FrameCenterServoHolder (Autodesk Fusion 360 design; units mm, degrees)
Autodesk Fusion 360 part; units mm, degrees
sketch "Sketch1" plane through (0, 0, 0) normal (0, 1, 0) x (1, 0, 0)
  line L0 (0, 26) -> (7, 26)
  line L1 (7, 26) -> (7, 6)
  line L2 (7, 6) -> (48, 6)
  line L3 (48, 6) -> (48, 26)
  line L4 (48, 26) -> (55, 26)
  line L5 (55, 26) -> (55, -9.8)
  line L6 (55, -9.8) -> (30.3, -9.8)
  line L7 (30.3, -9.8) -> (20.5, 0)
  line L8 (20.5, 0) -> (0, 0)
  line L9 (0, 26) -> (0, 0)
  line L10 (0, 0) -> (0, 39.3629) construction
  dimension "d1" = 7
  dimension "d2" = 7
  dimension "d3" = 41
  dimension "d4" = 6
  dimension "d5" = 15.8
  dimension "d7" = 135
  dimension "d8" = 20
  dimension "d98" = 20.5
  constraint perpendicular L0 L1
  constraint perpendicular L1 L2
  constraint perpendicular L2 L3
  constraint perpendicular L1 L4
  constraint perpendicular L4 L5
  constraint perpendicular L5 L6
  constraint collinear L0 L4
  constraint coincident L9.end L8
  constraint coincident L8.end L9.end
  constraint perpendicular L8 L9
  constraint vertical L10
  constraint collinear L9 L10
  measures "d1" distance of L0.start L0.end
  measures "d2" distance of L3.end L4.end
  measures "d3" distance of L1 L3
  measures "d4" distance of L2 L8
  measures "d5" distance of L2 L6
  measures "d7" angle of L6 L7
  measures "d8" distance of L2 L4
  measures "d98" distance of L7.end L8.end
extrude "Extrude1" add sketch "Sketch1" along normal blind 16
sketch "Sketch2" plane through (0, 16, 0) normal (0, 1, 0) x (-1, 0, 0)
  line L0 (-7, -26) -> (0, -26)
  line L1 (0, -26) -> (0, 0)
  line L2 (0, 0) -> (-20.5, 0)
  line L3 (-20.5, 0) -> (-30.3, 9.8)
  line L4 (-30.3, 9.8) -> (-55, 9.8)
  line L5 (-55, 9.8) -> (-55, -26)
  line L6 (-55, -26) -> (-48, -26)
  line L7 (-48, -26) -> (-48, -6)
  line L8 (-48, -6) -> (-7, -6)
  line L9 (-7, -6) -> (-7, -26)
  line L10 (-3, -22) -> (-52, -22) construction
  line L11 (-52, -22) -> (-52, -12) construction
  line L12 (-52, -12) -> (-3, -12) construction
  line L13 (-3, -12) -> (-3, -22) construction
  circle A0 centre (-3, -22) radius 1.75
  circle A1 centre (-3, -12) radius 1.75
  circle A2 centre (-52, -22) radius 1.75
  circle A3 centre (-52, -12) radius 1.75
  dimension "d11" = 3.5
  dimension "d12" = 3.5
  dimension "d13" = 3.5
  dimension "d14" = 3.5
  dimension "d15" = 49
  dimension "d16" = 10
  dimension "d17" = 55
  dimension "d18" = 20
  dimension "d19" = 4
  dimension "d20" = 3
  constraint horizontal L10
  constraint vertical L11
  constraint horizontal L12
  constraint vertical L13
  constraint coincident L10.start L13.end
  constraint coincident L12.end L13.start
  constraint coincident L10.end L11.start
  constraint coincident L11.end L12.start
  measures "d11" diameter of A0
  measures "d12" diameter of A1
  measures "d13" diameter of A2
  measures "d14" diameter of A3
  measures "d15" distance of L10.start L10.end
  measures "d16" distance of L10.start L12.end
  measures "d17" distance of L1 L5
  measures "d18" distance of L6.end L7.end
  measures "d19" distance of L6 L10
  measures "d20" distance of L1 L13
extrude "Extrude2" cut sketch "Sketch2" against normal up to surface (16 mm away) contours A0 | A1 | A2 | A3
ref_plane "WorkPlane1" through (27.5, 8, -8.1) normal (0, 1, 0) x (0, 0, 1)
ref_plane "WorkPlane2" through (27.5, 8, -16) normal (0, 0, -1) x (-1, 0, 0)
ref_plane "WorkPlane3" through (27.5, 8, -16) normal (-1, 0, 0) x (0, 0, 1)
ref_plane "WorkPlane4" through (27.5, 8, -8.1) normal (0, 1, 0) x (0, 0, 1)
sketch "Sketch3" plane through (27.5, 8, -7.6) normal (0, 1, 0) x (1, 0, 0)
  circle A0 centre (-24.5, 4.4) radius 1.75
  circle A1 centre (24.5, 14.4) radius 1.75
  circle A2 centre (-24.5, 14.4) radius 1.75
  circle A3 centre (24.5, 4.4) radius 1.75
  line L0 (-20.5, 18.4) -> (-27.5, 18.4)
  line L1 (-27.5, 18.4) -> (-27.5, -7.6)
  line L2 (-27.5, -7.6) -> (-7, -7.6)
  line L3 (-7, -7.6) -> (2.8, -17.4)
  line L4 (2.8, -17.4) -> (27.5, -17.4)
  line L5 (27.5, -17.4) -> (27.5, 18.4)
  line L6 (27.5, 18.4) -> (20.5, 18.4)
  line L7 (20.5, 18.4) -> (20.5, -1.6)
  line L8 (20.5, -1.6) -> (-20.5, -1.6)
  line L9 (-20.5, -1.6) -> (-20.5, 18.4)
  line L10 (-27.6177, 4.4) -> (-26.0588, 1.7)
  line L11 (-26.0588, 1.7) -> (-22.9412, 1.7)
  line L12 (-22.9412, 1.7) -> (-21.3823, 4.4)
  line L13 (-21.3823, 4.4) -> (-22.9412, 7.1)
  line L14 (-22.9412, 7.1) -> (-26.0588, 7.1)
  line L15 (-26.0588, 7.1) -> (-27.6177, 4.4)
  line L16 (-22.9412, 1.7) -> (-20.5, 1.7)
  line L17 (-26.0588, 1.7) -> (-27.5, 1.7)
  line L18 (-22.9412, 7.1) -> (-20.5, 7.1)
  line L19 (-26.0588, 7.1) -> (-27.5, 7.1)
  line L20 (-21.3823, 14.4) -> (-22.9412, 17.1)
  line L21 (-22.9412, 17.1) -> (-26.0588, 17.1)
  line L22 (-26.0588, 17.1) -> (-27.6177, 14.4)
  line L23 (-27.6177, 14.4) -> (-26.0588, 11.7)
  line L24 (-26.0588, 11.7) -> (-22.9412, 11.7)
  line L25 (-22.9412, 11.7) -> (-21.3823, 14.4)
  line L26 (-26.0588, 17.1) -> (-27.5, 17.1)
  line L27 (-26.0588, 11.7) -> (-27.5, 11.7)
  line L28 (-22.9412, 11.7) -> (-20.5, 11.7)
  line L29 (-22.9412, 17.1) -> (-20.5, 17.1)
  point P0 (-24.5, 4.4)
  point P1 (-24.5, 14.4)
  dimension "d23" = 5.4
  dimension "d88" = 5.4
  constraint coincident P0 A0.centre
  constraint parallel L2 L11
  constraint coincident L9 L16.end
  constraint perpendicular L9 L16
  constraint coincident L1 L17.end
  constraint perpendicular L1 L17
  constraint coincident L9 L18.end
  constraint perpendicular L9 L18
  constraint coincident L1 L19.end
  constraint perpendicular L1 L19
  constraint coincident P1 A2.centre
  constraint parallel L0 L21
  constraint coincident L1 L26.end
  constraint perpendicular L1 L26
  constraint coincident L1 L27.end
  constraint perpendicular L1 L27
  constraint coincident L9 L28.end
  constraint perpendicular L9 L28
  constraint coincident L9 L29.end
  constraint perpendicular L9 L29
  measures "d23" distance of L11 L14
  measures "d88" distance of L21 L24
extrude "Extrude3" cut sketch "Sketch3" along normal mid plane 2.5 contours L9 L20 L25 L28 L29 | L1 L22 L26 | L1 L20 L21 L22 L23 L24 L25 | L9 L12 L13 L16 L18 | L1 L23 L27 | L1 L10 L11 L12 L13 L14 L15 | L1 L15 L19 | L1 L10 L17
mirror "Mirror2" about plane through (27.5, 8, -16) normal (-1, 0, 0) of "Extrude3"
sketch "Sketch4" plane through (0, 16, 0) normal (0, 1, 0) x (-1, 0, 0)
  circle A0 centre (-3, -12) radius 1.75
  circle A1 centre (-52, -22) radius 1.75
  circle A2 centre (-3, -22) radius 1.75
  circle A3 centre (-52, -12) radius 1.75
  line L0 (-7, -26) -> (0, -26)
  line L1 (0, -26) -> (0, 0)
  line L2 (0, 0) -> (-20.5, 0)
  line L3 (-20.5, 0) -> (-30.3, 9.8)
  line L4 (-30.3, 9.8) -> (-55, 9.8)
  line L5 (-55, 9.8) -> (-55, -26)
  line L6 (-55, -26) -> (-48, -26)
  line L7 (-48, -26) -> (-48, -6)
  line L8 (-48, -6) -> (-7, -6)
  line L9 (-7, -6) -> (-7, -26)
  line L10 (-26.1569, 0) -> (-48, 0)
  line L11 (-48, 0) -> (-48, 5.8)
  line L12 (-48, 5.8) -> (-31.9569, 5.8)
  line L13 (-31.9569, 5.8) -> (-26.1569, 0)
  dimension "d30" = 4
  dimension "d31" = 4
  constraint parallel L2 L10
  constraint perpendicular L2 L11
  constraint perpendicular L11 L12
  constraint parallel L3 L13
  constraint collinear L2 L10
  constraint collinear L7 L11
  measures "d30" distance of L4 L12
  measures "d31" distance of L3 L13
extrude "Extrude4" cut sketch "Sketch4" against normal blind 16 contours L10 L11 L12 L13
sketch "Sketch5" plane through (55, 0, 0) normal (1, 0, 0) x (0, 0, -1)
  line L0 (14.7, 6.75) -> (9.3, 6.75)
  line L1 (9.3, 6.75) -> (9.3, 9.25)
  line L2 (9.3, 9.25) -> (14.7, 9.25)
  line L3 (14.7, 9.25) -> (14.7, 6.75)
  line L4 (-9.8, 0) -> (26, 0)
  line L5 (26, 0) -> (26, 16)
  line L6 (26, 16) -> (-9.8, 16)
  line L7 (-9.8, 16) -> (-9.8, 0)
  line L8 (-5.8, 16) -> (0, 16)
  line L9 (0, 16) -> (0, 0)
  line L10 (0, 0) -> (-5.8, 0)
  line L11 (-5.8, 0) -> (-5.8, 16)
  line L12 (10.25, 16) -> (13.75, 16)
  line L13 (10.25, 9.25) -> (13.75, 9.25)
  line L14 (20.25, 16) -> (23.75, 16)
  line L15 (13.75, 6.75) -> (10.25, 6.75)
  line L16 (13.75, 0) -> (10.25, 0)
  line L17 (23.75, 0) -> (20.25, 0)
  line L18 (6, 0) -> (6, 16)
  line L19 (6, 16) -> (6, 0)
  line L20 (-9.8, 8) -> (26, 8) construction
  circle A0 centre (-2.9, 8) radius 1.75
  line L21 (17, 16) -> (17, 0) construction
  circle A1 centre (17, 12) radius 1.75
  circle A2 centre (17, 4) radius 1.75
  line L22 (24.7, 6.75) -> (19.3, 6.75)
  line L23 (19.3, 6.75) -> (19.3, 9.25)
  line L24 (19.3, 9.25) -> (24.7, 9.25)
  line L25 (24.7, 9.25) -> (24.7, 6.75)
  line L26 (20.25, 9.25) -> (23.75, 9.25)
  line L27 (23.75, 6.75) -> (20.25, 6.75)
  line L28 (12, 16) -> (12, 0) construction
  line L29 (22, 16) -> (22, 0) construction
  dimension "d34" = 3.5
  dimension "d35" = 5.8
  dimension "d36" = 2.9
  dimension "d37" = 20
  dimension "d39" = 3.5
  dimension "d40" = 3.5
  dimension "d41" = 16
  dimension "d42" = 4
  dimension "d43" = 4
  dimension "d90" = 10
  dimension "d91" = 5
  constraint midpoint L7 L20.start
  constraint midpoint L5 L20.end
  constraint coincident L20 A0.centre
  constraint coincident L6 L21.start
  constraint coincident L4 L21.end
  constraint perpendicular L4 L21
  constraint coincident L21 A1.centre
  constraint coincident L21 A2.centre
  constraint midpoint L12 L28.start
  constraint midpoint L16 L28.end
  constraint midpoint L14 L29.start
  constraint midpoint L17 L29.end
  measures "d34" diameter of A0
  measures "d35" distance of L9 L11
  measures "d36" distance of L11 A0.centre
  measures "d37" distance of L5 L18
  measures "d39" diameter of A1
  measures "d40" diameter of A2
  measures "d41" distance of L4.end L5.end
  measures "d42" distance of L6 A1.centre
  measures "d43" distance of L4 A2.centre
  measures "d90" distance of L28 L29
  measures "d91" distance of L21 L28
extrude "Extrude5" cut sketch "Sketch5" against normal up to surface (7 mm away) contours A0 | A1 | A2
sketch "Sketch6" plane through (48, 0, 0) normal (-1, 0, 0) x (0, 0, 1)
  circle A0 centre (-17, 12) radius 1.75
  circle A1 centre (-17, 4) radius 1.75
  line L0 (-9.3, 6.75) -> (-14.7, 6.75)
  line L1 (-14.7, 6.75) -> (-14.7, 9.25)
  line L2 (-14.7, 9.25) -> (-9.3, 9.25)
  line L3 (-9.3, 9.25) -> (-9.3, 6.75)
  line L4 (-26, 0) -> (-6, 0)
  line L5 (-6, 0) -> (-6, 16)
  line L6 (-6, 16) -> (-26, 16)
  line L7 (-26, 16) -> (-26, 0)
  circle A2 centre (-17, 4) radius 2.9
  circle A3 centre (-17, 12) radius 2.9
  line L8 (-19.3, 6.75) -> (-24.7, 6.75)
  line L9 (-24.7, 6.75) -> (-24.7, 9.25)
  line L10 (-24.7, 9.25) -> (-19.3, 9.25)
  line L11 (-19.3, 9.25) -> (-19.3, 6.75)
  circle A4 centre (2.9, 8) radius 1.75
  line L12 (5.8, 16) -> (0, 16)
  line L13 (0, 16) -> (0, 0)
  line L14 (0, 0) -> (5.8, 0)
  line L15 (5.8, 0) -> (5.8, 16)
  circle A5 centre (2.9, 8) radius 2.9
  dimension "d46" = 5.8
  dimension "d47" = 5.8
  dimension "d89" = 5.8
  constraint concentric A1 A2
  constraint concentric A0 A3
  constraint concentric A4 A5
  measures "d46" diameter of A2
  measures "d47" diameter of A3
  measures "d89" diameter of A5
extrude "Extrude6" cut sketch "Sketch6" against normal blind 3 contours A2 | A3 | A5
sketch "Sketch7" plane through (0, 0, 0) normal (-1, 0, 0) x (0, 0, 1)
  line L0 (-9.3, 6.75) -> (-14.7, 6.75)
  line L1 (-14.7, 6.75) -> (-14.7, 9.25)
  line L2 (-14.7, 9.25) -> (-9.3, 9.25)
  line L3 (-9.3, 9.25) -> (-9.3, 6.75)
  line L4 (-26, 0) -> (0, 0)
  line L5 (0, 0) -> (0, 16)
  line L6 (0, 16) -> (-26, 16)
  line L7 (-26, 16) -> (-26, 0)
  line L8 (0, 0) -> (9.8, 0)
  line L9 (9.8, 0) -> (9.8, 16)
  line L10 (9.8, 16) -> (0, 16)
  line L11 (0, 16) -> (0, 0)
  line L12 (0, 13) -> (5, 13)
  line L13 (5, 13) -> (5, 3)
  line L14 (5, 3) -> (0, 3)
  line L15 (0, 3) -> (0, 13)
  line L16 (-19.3, 6.75) -> (-24.7, 6.75)
  line L17 (-24.7, 6.75) -> (-24.7, 9.25)
  line L18 (-24.7, 9.25) -> (-19.3, 9.25)
  line L19 (-19.3, 9.25) -> (-19.3, 6.75)
  circle A0 centre (2.9, 8) radius 2.9
  circle A1 centre (2.9, 8) radius 1.75
  dimension "d50" = 5
  dimension "d51" = 10
  dimension "d52" = 16
  dimension "d53" = 3
  constraint horizontal L12
  constraint vertical L13
  constraint horizontal L14
  constraint vertical L15
  constraint coincident L5 L12.start
  measures "d50" distance of L13 L15
  measures "d51" distance of L12.end L13.end
  measures "d52" distance of L8.end L9.end
  measures "d53" distance of L10 L12
extrude "Extrude7" cut sketch "Sketch7" along normal up to surface contours L5 L11 L13 L14 L15 A0 | L5 L11 L12 L13 L15 A0 | L13 A0 | L13 A0 | A1 end surface through (31.9569, 16, 5.8) normal (0.707107, 0, -0.707107) offset 0
sketch "Sketch8" plane through (27.5, 8, -7.6) normal (0, 1, 0) x (1, 0, 0)
  line L0 (20.5, -7.6) -> (20.5, -13.4)
  line L1 (20.5, -13.4) -> (4.4569, -13.4)
  circle A0 centre (-24.5, 4.4) radius 1.75
  circle A1 centre (24.5, 14.4) radius 1.75
  circle A2 centre (-24.5, 14.4) radius 1.75
  circle A3 centre (24.5, 4.4) radius 1.75
  line L2 (-20.5, 18.4) -> (-27.5, 18.4)
  line L3 (-27.5, 18.4) -> (-27.5, -7.6)
  line L4 (-1.3431, -7.6) -> (20.5, -7.6)
  line L5 (2.8, -17.4) -> (27.5, -17.4)
  line L6 (27.5, -17.4) -> (27.5, 18.4)
  line L7 (27.5, 18.4) -> (20.5, 18.4)
  line L8 (20.5, 18.4) -> (20.5, -1.6)
  line L9 (20.5, -1.6) -> (-20.5, -1.6)
  line L10 (-20.5, -1.6) -> (-20.5, 18.4)
  line L11 (20.5, -7.6) -> (27.5, -7.6)
  line L12 (27.5, -2.6) -> (13.5, -2.6)
  line L13 (13.5, -2.6) -> (4.8397, -7.6)
  line L14 (4.4569, -13.4) -> (-1.3431, -7.6)
  line L15 (-7, -7.6) -> (2.8, -17.4)
  line L16 (-27.5, -7.6) -> (-7, -7.6)
  dimension "d56" = 5
  dimension "d57" = 150
  dimension "d99" = 7
  dimension "d100" = 14
  constraint coincident L0.start L4.end
  constraint coincident L6 L11.end
  constraint perpendicular L6 L11
  constraint coincident L6 L12.start
  constraint perpendicular L6 L12
  constraint coincident L4 L13.end
  measures "d56" distance of L11 L12
  measures "d57" angle of L12 L13
  measures "d99" distance of L0.start L11.end
  measures "d100" distance of L12.start L12.end
extrude "Extrude8" cut sketch "Sketch8" along normal mid plane 10 contours L4 L6 L11 L12 L13
sketch "Sketch13" plane through (48, 0, 0) normal (-1, 0, 0) x (0, 0, 1)
  circle A0 centre (-17, 4) radius 2.9
  circle A1 centre (-17, 12) radius 2.9
  line L0 (-9.3, 6.75) -> (-14.7, 6.75)
  line L1 (-14.7, 6.75) -> (-14.7, 9.25)
  line L2 (-14.7, 9.25) -> (-9.3, 9.25)
  line L3 (-9.3, 9.25) -> (-9.3, 6.75)
  line L4 (-26, 0) -> (-6, 0)
  line L5 (-6, 0) -> (-6, 16)
  line L6 (-6, 16) -> (-26, 16)
  line L7 (-26, 16) -> (-26, 0)
  line L8 (-19.3, 6.75) -> (-24.7, 6.75)
  line L9 (-24.7, 6.75) -> (-24.7, 9.25)
  line L10 (-24.7, 9.25) -> (-19.3, 9.25)
  line L11 (-19.3, 9.25) -> (-19.3, 6.75)
  point P0 (-24, 16)
  point P1 (-26, 14)
  dimension "d81" = 2
  dimension "d82" = 2
  constraint coincident L6 P0
  constraint coincident L7 P1
  measures "d81" distance of L7 P0
  measures "d82" distance of L6 P1
sketch "Sketch14" plane through (0, 0, -26) normal (0, 0, -1) x (-1, 0, 0)
  line L0 (-55, 0) -> (-48, 0)
  line L1 (-48, 0) -> (-48, 16)
  line L2 (-48, 16) -> (-55, 16)
  line L3 (-55, 16) -> (-55, 0)
  point P0 (-50, 16)
  dimension "d83" = 2
  constraint coincident L2 P0
  measures "d83" distance of L1 P0
ref_plane "WorkPlane6" through (50, 16, -26) normal (0.57735, -0.57735, 0.57735) x (0.707107, 0.707107, 0)
sketch "Sketch15" plane through (50, 16, -26) normal (0.57735, -0.57735, 0.57735) x (0.712442, 0.701648, -0.010795)
  line L0 (-2.8282, -0.0374) -> (0, 0)
  line L1 (0, 0) -> (-1.4465, 2.4306)
  line L2 (-1.4465, 2.4306) -> (-2.8282, -0.0374)
  point P0 (-1.4465, 2.4306)
  point P1 (-2.8282, -0.0374)
  constraint coincident P1 L0.start
  constraint coincident L0.end L1.start
  constraint coincident P0 L1.end
extrude "Extrude11" cut sketch "Sketch15" against normal up to surface (1.1547 mm away)
mirror "Mirror4" about plane through (27.5, 8, -8.1) normal (0, 1, 0) of "Extrude11"
sketch "Sketch16" plane through (0, 0, 0) normal (-1, 0, 0) x (0, 0, 1)
  line L0 (-9.3, 6.75) -> (-14.7, 6.75)
  line L1 (-14.7, 6.75) -> (-14.7, 9.25)
  line L2 (-14.7, 9.25) -> (-9.3, 9.25)
  line L3 (-9.3, 9.25) -> (-9.3, 6.75)
  line L4 (-19.3, 6.75) -> (-24.7, 6.75)
  line L5 (-24.7, 6.75) -> (-24.7, 9.25)
  line L6 (-24.7, 9.25) -> (-19.3, 9.25)
  line L7 (-19.3, 9.25) -> (-19.3, 6.75)
  line L8 (-26, 0) -> (0, 0)
  line L9 (0, 0) -> (0, 16)
  line L10 (0, 16) -> (-26, 16)
  line L11 (-26, 16) -> (-26, 0)
  line L12 (0, 13) -> (5, 13)
  line L13 (5, 13) -> (5, 10)
  arc A0 (5, 6) -> (5, 10) centre (2.9, 8) ccw
  line L14 (5, 6) -> (5, 3)
  line L15 (5, 3) -> (0, 3)
  line L16 (0, 3) -> (0, 0)
  line L17 (0, 0) -> (9.8, 0)
  line L18 (9.8, 0) -> (9.8, 16)
  line L19 (9.8, 16) -> (0, 16)
  line L20 (0, 16) -> (0, 13)
  line L21 (0, 3) -> (-2, 5)
  line L22 (-2, 5) -> (-2, 11)
  line L23 (-2, 11) -> (0, 13)
  dimension "d93" = 45
  dimension "d94" = 45
  dimension "d95" = 2
  constraint coincident L15.end L16.start
  constraint perpendicular L15 L22
  constraint coincident L12.start L20.end
  measures "d93" angle of L9 L21
  measures "d94" angle of L9 L23
  measures "d95" distance of L9 L22
extrude "Extrude12" cut sketch "Sketch16" along normal up to surface contours L9 L21 L22 L23 end surface through (41, 8, -5) normal (0.5, 0, 0.866025) offset 0
sketch "Sketch9" plane through (0, 0, 0) normal (-1, 0, 0) x (0, 0, 1)
  line L0 (-26, 16) -> (-26, 0)
  line L1 (-9.3, 6.75) -> (-14.7, 6.75)
  line L2 (-14.7, 6.75) -> (-14.7, 9.25)
  line L3 (-14.7, 9.25) -> (-9.3, 9.25)
  line L4 (-9.3, 9.25) -> (-9.3, 6.75)
  line L5 (-9.3, 6.75) -> (-14.7, 6.75)
  line L6 (-14.7, 6.75) -> (-14.7, 9.25)
  line L7 (-14.7, 9.25) -> (-9.3, 9.25)
  line L8 (-9.3, 9.25) -> (-9.3, 6.75)
  circle A0 centre (-17, 12) radius 2.9
  circle A1 centre (-17, 4) radius 2.9
  line L9 (-6, 0) -> (-6, 16)
  circle A2 centre (-17, 12) radius 1.75
  circle A3 centre (-17, 4) radius 1.75
  circle A4 centre (-17, 12) radius 2.5
  circle A5 centre (-17, 4) radius 2.5
  line L10 (-24, 16) -> (-26, 14)
  line L11 (-26, 2) -> (-24, 0)
  line L12 (-24.7, 6.75) -> (-24.7, 9.25)
  line L13 (-19.3, 9.25) -> (-19.3, 6.75)
  line L14 (-24.7, 6.75) -> (-24.7, 9.25)
  line L15 (-19.3, 9.25) -> (-19.3, 6.75)
  line L16 (-19.3, 6.75) -> (-24.7, 6.75)
  line L17 (-24.7, 9.25) -> (-19.3, 9.25)
  line L18 (0, 3) -> (-2, 5)
  line L19 (-2, 5) -> (-2, 11)
  line L20 (-2, 11) -> (0, 13)
  line L21 (0, 13) -> (0, 16)
  line L22 (0, 16) -> (-26, 16)
  line L23 (-26, 0) -> (0, 0)
  line L24 (0, 0) -> (0, 3)
  line L25 (-24, 0) -> (-6, 0)
  line L26 (-6, 16) -> (-24, 16)
  line L27 (-26, 14) -> (-26, 2)
  line L28 (-19.3, 6.75) -> (-24.7, 6.75)
  line L29 (-24.7, 9.25) -> (-19.3, 9.25)
  dimension "d67" = 5
  dimension "d68" = 5
  constraint concentric A2 A4
  constraint concentric A3 A5
  measures "d67" diameter of A4
  measures "d68" diameter of A5
extrude "Extrude9" cut sketch "Sketch9" against normal up to surface (7 mm away) contours A2 | A3 | A4 | A5
chamfer "Chamfer1" distance 5 angle 45 2 edges at (0, 14.5, 0) (0, 1.5, 0)
chamfer "Chamfer5" distance 0.5 angle 45 4 edges at (48, 0, 2.9) (39.9784, 0, 5.8) (29.0569, 0, 2.9) (37.0784, 0, 0)
chamfer "Chamfer6" distance 1.5 angle 45 4 edges at (48, 16, 2.9) (39.9784, 16, 5.8) (29.0569, 16, 2.9) (37.0784, 16, 0)
chamfer "Chamfer7" distance 2 angle 45 8 edges at (2.5, 0, -2.5) (12.75, 0, 0) (25.4, 0, 4.9) (42.65, 0, 9.8) (42.65, 16, 9.8) (25.4, 16, 4.9) (12.75, 16, 0) (2.5, 16, -2.5)
chamfer "Chamfer8" distance 0.5 angle 45 7 edges at (55, 16, -9.1) (52.5, 16, -26) (48, 16, -15) (27.5, 16, -6) (7, 16, -16) (3.5, 16, -26) (0, 16, -16.9142)
chamfer "Chamfer8" distance 0.5 angle 45 1 edges at (48, 8, -26)
chamfer "Chamfer9" distance 0.5 angle 45 7 edges at (0, 0, -16.9142) (3.5, 0, -26) (7, 0, -16) (27.5, 0, -6) (48, 0, -16) (51.5, 0, -26) (55, 0, -9.1)
equation "d2 = d1"
equation "d12 = d11"
equation "d13 = d11"
equation "d14 = d11"
equation "d19 = ( d18 - d16 ) / 2 - 1 mm"
equation "d20 = ( d17 - d15 ) / 2"
equation "d31 = d30"
equation "d36 = d35 / 2"
equation "d39 = d34"
equation "d40 = d34"
equation "d42 = d41 / 4"
equation "d43 = d42"
equation "d47 = d46"
equation "d53 = ( d52 - d51 ) / 2"
equation "d68 = d67"
equation "d82 = d81"
equation "d88 = d23"
equation "d89 = d46"
equation "d91 = d90 / 2"
equation "d94 = d93"
equation "d100 = d99 * 2"
